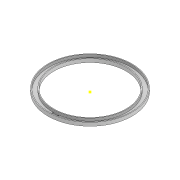
# Autodesk Inventor part: led_ring
Saved by Autodesk Inventor 2020 (Build 240168000, 168)
## iProperties
Created: 2020-05-05
Part Number: led_ring
Material: Generic
Document SubType Name: Modeling
Designer: User
Density: 1 g/cm^3
Appearance: Default
Author: User
Autodesk Inventor part; units mm, degrees
ref_plane "YZ Plane" through (0, 0, 0) normal (1, 0, 0) x (0, 1, 0)
ref_plane "XZ Plane" through (0, 0, 0) normal (0, 1, 0) x (-1, 0, 0)
ref_plane "XY Plane" through (0, 0, 0) normal (0, 0, 1) x (1, 0, 0)
sketch "Sketch1" plane through (0, 0, 0) normal (0, 1, 0) x (-1, 0, 0)
  point P0 (0, 0)
sketch "Sketch2" plane through (0, 0, 0) normal (0, 1, 0) x (-1, 0, 0)
  circle A0 centre (0, 0) radius 79.375
  circle A1 centre (0, 0) radius 71.12
  dimension "d0" = 158.75
  dimension "d1" = 142.24
  constraints: 2 centre point, 2 coincident
  measures "d0" diameter of A0
  measures "d1" diameter of A1
extrude "Extrusion1" add sketch "Sketch2" along normal blind 1.5875
sketch "Sketch3" plane through (0, 1.5875, 0) normal (0, 1, 0) x (1, 0, 0)
  circle A0 centre (0, 0) radius 80.9625
  circle A1 centre (0, 0) radius 69.5325
  circle A2 centre (0, 0) radius 71.12 projected
  circle A3 centre (0, 0) radius 79.375 projected
  circle A4 centre (0, 0) radius 79.375 projected
  circle A5 centre (0, 0) radius 71.12 projected
  dimension "d4" = 1.5875
  dimension "d5" = 1.5875
  constraints: 2 centre point, 2 coincident
  measures "d4" radial gap between concentric circles of A1 A2
  measures "d5" radial gap between concentric circles of A3 A0
extrude "Extrusion2" add sketch "Sketch3" along normal blind 5 and the other way blind 1.5875
sketch "Sketch4" plane through (0, 1.5875, 0) normal (0, 1, 0) x (1, 0, 0)
  circle A0 centre (0, 0) radius 79.375 projected
  circle A1 centre (0, 0) radius 71.12 projected
  circle A2 centre (0, 0) radius 71.12 projected
  line L0 (0, -71.12) -> (0, -79.375)
  circle A3 centre (0, 0) radius 80.9625 projected
  line L1 (0, 0) -> (12.4554, -78.3917)
  point P0 (11.16, -70.2389)
  constraints: 4 end point, 2 point on circle, 1 vertical, 1 vertical alignment, 1 other
extrude "Extrusion3" cut sketch "Sketch4" against normal blind 5 contours L0 A1 L1 A0 picked at (10.6461, -75.856)
fillet "Fillet1" radius 1.5875 4 edges at (11.16, 0.7937, 70.2389) (12.4554, 0.7937, 78.3917) (0, 0.7937, 79.375) (0, 0.7937, 71.12)
body "Solid1"
